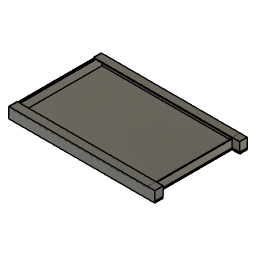
porte carte v3 (Autodesk Fusion 360 design; units mm, degrees)
Autodesk Fusion 360 part; units mm, degrees
sketch "Esquisse1" plane through (0, 0, 0) normal (0, 0, 1) x (1, 0, 0)
  line L0 (0, 0) -> (85, 0)
  line L1 (85, 0) -> (85, 55)
  line L2 (85, 55) -> (0, 55)
  line L3 (0, 55) -> (0, 0)
  dimension "d1" = 85
  dimension "d2" = 55
  constraint horizontal L0
  constraint vertical L1
  constraint horizontal L2
  constraint vertical L3
  constraint coincident L0.start L3.end
  measures "d1" distance of L0.start L0.end
  measures "d2" distance of L0.start L2.end
sketch "Esquisse2" plane through (0, 0, 0) normal (0, 0, 1) x (1, 0, 0)
  line L0 (-2, -2) -> (87, -2)
  line L1 (87, -2) -> (87, 57)
  line L2 (87, 57) -> (-2, 57)
  line L3 (-2, 57) -> (-2, -2)
  line L4 (0, 0) -> (85, 0)
  line L5 (85, 55) -> (0, 55)
  line L6 (85, 0) -> (85, 55)
  line L7 (0, 55) -> (0, 0)
  line L8 (87.5, -2.5) -> (87.5, 57.5)
  line L9 (87.5, 57.5) -> (-2.5, 57.5)
  line L10 (-2.5, 57.5) -> (-2.5, -2.5)
  line L11 (-2.5, -2.5) -> (87.5, -2.5)
  dimension "d3" = 2
  dimension "d4" = 2
  dimension "d5" = 2
  dimension "d6" = 2
  dimension "d7" = 0.5
  constraint horizontal L0
  constraint vertical L1
  constraint horizontal L2
  constraint vertical L3
  measures "d3" distance of L0 L4
  measures "d4" distance of L2 L5
  measures "d5" distance of L1 L6
  measures "d6" distance of L3 L7
extrude "Extrusion1" add sketch "Esquisse2" along normal blind 5 contours L4 L5 L6 L7 makes body 1
extrude "Extrusion2" add sketch "Esquisse2" against normal blind 0.5 separate body contours L0 L1 L2 L3 makes body 2
extrude "Extrusion3" add sketch "Esquisse2" along normal blind 5.5 and the other way blind 0.5 contours L8 L9 L10 L11 bodies 2
extrude "Extrusion4" add 1 faces at (85, 18.3333, -0.1667) along direction (-1, 0, 0) blind 85 on bodies 2 bodies 2
sketch "Esquisse3" plane through (0, 0, 5.5) normal (0, 0, 1) x (-1, 0, 0)
  line L0 (2, 2) -> (2, -57)
  line L1 (2, -57) -> (-87, -57)
  line L2 (-87, -57) -> (-87, 2)
  line L3 (-87, 2) -> (2, 2)
  line L4 (2.5, 2.5) -> (-87.5, 2.5)
  line L5 (-87.5, 2.5) -> (-87.5, -57.5)
  line L6 (-87.5, -57.5) -> (2.5, -57.5)
  line L7 (2.5, -57.5) -> (2.5, 2.5)
  line L8 (2.5, 2.5) -> (-87.5, 2.5)
  line L9 (-87.5, 2.5) -> (-87.5, -57.5)
  line L10 (-87.5, -57.5) -> (2.5, -57.5)
  line L11 (2.5, -57.5) -> (2.5, 2.5)
  dimension "d18" = 60
  dimension "d19" = 90
  constraint horizontal L8
  constraint vertical L9
  constraint horizontal L10
  constraint vertical L11
  constraint coincident L4.start L7.end
  measures "d18" distance of L4.end L5.end
  measures "d19" distance of L5.end L6.end
extrude "Extrusion5" add sketch "Esquisse3" along normal blind 0.5 separate body contours L0 L1 L2 L3 makes body 3
extrude "Extrusion6" add 1 faces at (-2, 17.6667, 5.6667) along direction (-1, 0, 0) blind 0.5 on bodies 3 bodies 3
extrude "Extrusion7" add 1 faces at (27.3333, 57, 5.8333) along direction (0, 1, 0) blind 0.5 on bodies 3 bodies 3
extrude "Extrusion8" add 1 faces at (87, 37.6667, 5.8333) along direction (1, 0, 0) blind 0.5 on bodies 3 bodies 3
extrude "Extrusion9" add 1 faces at (27.5, -2, 5.6667) along direction (0, -1, 0) blind 0.5 on bodies 3 bodies 3
sketch "Esquisse4" plane through (87.5, 0, 0) normal (1, 0, 0) x (0, 1, 0)
  line L0 (57.5, -0.5) -> (57.5, 5.5)
  line L1 (57.5, 5.5) -> (-2.5, 5.5)
  line L2 (-2.5, 5.5) -> (-2.5, -0.5)
  line L3 (-2.5, -0.5) -> (57.5, -0.5)
  line L4 (-2, 0.5) -> (57, 0.5)
  line L5 (57, 0.5) -> (57, 0)
  line L6 (57, 0) -> (-2, 0)
  line L7 (-2, 0) -> (-2, 0.5)
  line L8 (-2.5, -0.5) -> (2.5, -0.5)
  line L9 (2.5, -0.5) -> (2.5, 4.5)
  line L10 (2.5, 4.5) -> (-2.5, 4.5)
  line L11 (-2.5, 4.5) -> (-2.5, -0.5)
  line L12 (57.5, -0.5) -> (52.5, -0.5)
  line L13 (52.5, -0.5) -> (52.5, 4.5)
  line L14 (52.5, 4.5) -> (57.5, 4.5)
  line L15 (57.5, 4.5) -> (57.5, -0.5)
  dimension "d30" = 0.5
  dimension "d31" = 0.5
  dimension "d32" = 0.5
  dimension "d33" = 0.5
  dimension "d34" = 5
  dimension "d35" = 5
  dimension "d36" = 5
  dimension "d37" = 5
  constraint horizontal L4
  constraint vertical L5
  constraint horizontal L6
  constraint vertical L7
  constraint horizontal L8
  constraint vertical L9
  constraint horizontal L10
  constraint vertical L11
  constraint coincident L2.end L3.start
  constraint horizontal L12
  constraint vertical L13
  constraint horizontal L14
  constraint vertical L15
  constraint coincident L0.start L3.end
  measures "d30" distance of L3 L6
  measures "d31" distance of L2 L7
  measures "d32" distance of L0 L5
  measures "d33" distance of L4 L6
  measures "d34" distance of L2.end L8.end
  measures "d35" distance of L2.end L10.end
  measures "d36" distance of L0.start L12.end
  measures "d37" distance of L0.start L14.end
extrude "Extrusion10" add sketch "Esquisse4" along normal blind 5 contours L2 L3 L4 L6 L7 L8 L9 L10 L11 bodies 2
extrude "Extrusion11" add sketch "Esquisse4" along normal blind 5 contours L0 L3 L4 L5 L6 L12 L13 L14 L15 bodies 2
extrude "Extrusion12" cut sketch "Esquisse4" against normal blind 1 contours L4 L6 L9 L13 bodies 2
extrude "Extrusion13" cut 1 faces at (87.3333, 2.5, 0.1667) along direction (0, -1, 0) blind 4.5 on bodies 2 bodies 2
extrude "Extrusion14" cut 1 faces at (87.3333, 52.5, 0.1667) along direction (0, 1, 0) blind 4.5 on bodies 2 bodies 2
extrude "Extrusion15" add 1 faces at (89.1667, 0.8333, 4.5) along direction (0, 0, 1) blind 1 on bodies 2 bodies 2
extrude "Extrusion16" add 1 faces at (89.1667, 54.1667, 4.5) along direction (0, 0, 1) blind 1 on bodies 2 bodies 2
extrude "Extrusion17" add 1 faces at (90.8333, 0.8333, 5.5) along direction (0, 0, 1) blind 0.5 on bodies 2 bodies 2
extrude "Extrusion18" add 1 faces at (60.8333, -2.5, 3.8333) along direction (0, -1, 0) blind 0.5 on bodies 2 bodies 2
extrude "Extrusion19" add 1 faces at (-2.5, 17.1667, 3.8333) along direction (-1, 0, 0) blind 0.5 on bodies 2 bodies 2
sketch "Esquisse5" plane through (0, 0, 6) normal (0, 0, 1) x (-1, 0, 0)
  line L0 (2, 2) -> (2, -57)
  line L1 (2, -57) -> (-87, -57)
  line L2 (-87, -57) -> (-87, 2)
  line L3 (-87, 2) -> (2, 2)
  line L4 (-92.5, 3) -> (-92.5, -2.5)
  line L5 (-92.5, -2.5) -> (-87.5, -2.5)
  line L6 (-87.5, -2.5) -> (-87.5, -52.5)
  line L7 (-87.5, -52.5) -> (-92.5, -52.5)
  line L8 (-92.5, -52.5) -> (-92.5, -57.5)
  line L9 (-92.5, -57.5) -> (3, -57.5)
  line L10 (3, -57.5) -> (3, 3)
  line L11 (3, 3) -> (-92.5, 3)
  line L12 (-87.5, 3) -> (3, 3)
  line L13 (3, 3) -> (3, -2.5)
  line L14 (3, -2.5) -> (-87.5, -2.5)
  line L15 (-87.5, -2.5) -> (-87.5, 3)
  line L16 (3, -57.5) -> (-87.5, -57.5)
  line L17 (-87.5, -57.5) -> (-87.5, -52.5)
  line L18 (-87.5, -52.5) -> (3, -52.5)
  line L19 (3, -52.5) -> (3, -57.5)
  dimension "d58" = 5.5
  constraint coincident L11 L12.start
  constraint horizontal L12
  constraint vertical L13
  constraint horizontal L14
  constraint vertical L15
  constraint coincident L10 L13.end
  constraint horizontal L16
  constraint vertical L17
  constraint horizontal L18
  constraint vertical L19
  constraint coincident L6.end L7.start
  constraint coincident L9.end L10.start
  measures "d58" distance of L12 L14
extrude "Extrusion20" add sketch "Esquisse5" along normal blind 0.5 contours L0 L2 L3 L10 L11 L12 L13 L14 L15 | L0 L2 L3 L14 bodies 2
extrude "Extrusion21" add 1 faces at (89.1667, -1.1667, 6) along direction (0, 0, 1) blind 0.5 on bodies 2 bodies 2
extrude "Extrusion22" add sketch "Esquisse5" along normal blind 0.5 contours L0 L1 L2 L9 L10 L16 L17 L18 L19 | L0 L1 L2 L18 bodies 2
extrude "Extrusion23" add sketch "Esquisse5" along normal blind 0.5 contours L7 L8 L9 L17 bodies 2
sketch "Esquisse6" plane through (0, 57.5, 0) normal (0, 1, 0) x (-1, 0, 0)
  line L0 (-92.5, 6.5) -> (-92.5, -0.5)
  line L1 (-92.5, -0.5) -> (3, -0.5)
  line L2 (3, -0.5) -> (3, 6.5)
  line L3 (3, 6.5) -> (-92.5, 6.5)
  line L4 (2.5, 6) -> (-87.5, 6)
  line L5 (-87.5, 6) -> (-87.5, 5.5)
  line L6 (-87.5, 5.5) -> (2.5, 5.5)
  line L7 (2.5, 5.5) -> (2.5, 6)
  dimension "d67" = 90
  dimension "d68" = 0.5
  dimension "d69" = 0.5
  dimension "d70" = 0.5
  constraint horizontal L4
  constraint vertical L5
  constraint horizontal L6
  constraint vertical L7
  measures "d67" distance of L4.start L4.end
  measures "d68" distance of L4.end L5.end
  measures "d69" distance of L3 L4
  measures "d70" distance of L2 L7
extrude "Extrusion24" cut sketch "Esquisse6" against normal blind 60 contours L4 L5 L6 L7 bodies 2
hidden bodies 1 3
